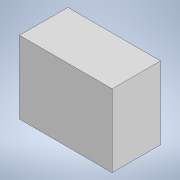
# Autodesk Inventor part: peg_TL
Saved by Autodesk Inventor 2020 (Build 240168000, 168)
## iProperties
Created: 2019-07-24
Part Number: peg_TL
Material: Generic
Document SubType Name: Modeling
Designer: Dammy
Density: 1 g/cm^3
Appearance: Default
Author: Dammy
Autodesk Inventor part; units mm, degrees
ref_plane "YZ Plane" through (0, 0, 0) normal (1, 0, 0) x (0, 1, 0)
ref_plane "XZ Plane" through (0, 0, 0) normal (0, 1, 0) x (-1, 0, 0)
ref_plane "XY Plane" through (0, 0, 0) normal (0, 0, 1) x (1, 0, 0)
sketch "base" plane through (0, 0, 0) normal (0, 1, 0) x (-1, 0, 0)
  line L0 (-11.5, 6) -> (11.5, 6)
  line L1 (11.5, 6) -> (11.5, -6)
  line L2 (11.5, -6) -> (-11.5, -6)
  line L3 (-11.5, -6) -> (-11.5, 6)
  line L4 (-11.5, 6) -> (11.5, -6) construction
  line L5 (11.5, 6) -> (-11.5, -6) construction
  point P0 (0, 0)
  dimension "d0" = 23
  dimension "d1" = 12
  constraints: 12 end point, 2 midpoint, 2 parallel, 1 horizontal, 1 perpendicular
  measures "d0" distance of L1.end L2.end
  measures "d1" distance of L0.end L1.end
extrude "Extrusion1" add sketch "base" along normal blind 18
sketch "Sketch2" plane through (11.5, 0, -6) normal (0, 0, -1) x (-1, 0, 0)
  line L0 (23, 15) -> (3, 15)
  line L1 (3, 15) -> (3, 9.9)
  line L2 (3, 9.9) -> (23, 9.9)
  line L3 (23, 9.9) -> (23, 15)
  line L4 (23, 0) -> (23, 18) projected
  line L5 (0, 18) -> (23, 18) projected
  line L6 (0, 0) -> (0, 18) projected
  point P0 (11.5, 0)
  dimension "d4" = 3
  dimension "d5" = 5.1
  dimension "d6" = 3
  constraints: 8 end point, 2 parallel, 1 horizontal, 1 perpendicular, 1 point on line
  measures "d4" distance between parallel lines of L5 L0
  measures "d5" distance between parallel lines of L2 L0
  measures "d6" distance between parallel lines of L6 L1
extrude "Extrusion2" cut sketch "Sketch2" against normal blind 9
equation "\"d6\" = d4"
body "Solid1"
